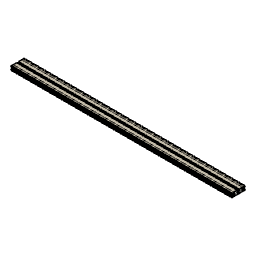
vector rail profile (Autodesk Fusion 360 design; units mm, degrees)
Autodesk Fusion 360 part; units mm, degrees
sketch "Sketch1" plane through (0, 0, 0) normal (1, 0, 0) x (0, 0, -1)
  line L0 (-12.7, -4.6736) -> (-12.7, -2.4765)
  line L1 (-12.7, -2.4765) -> (-10.8458, -2.4765)
  line L2 (-10.8458, -2.4765) -> (-10.8458, -3.556)
  line L3 (-10.8458, -3.556) -> (-8.2042, -3.556)
  line L4 (-8.2042, -3.556) -> (-8.2042, -2.4765)
  line L5 (-8.2042, -2.4765) -> (-6.9342, -2.4765)
  line L6 (-6.9342, -2.4765) -> (-6.9342, 0.5207)
  line L7 (-6.9342, 0.5207) -> (-8.2042, 0.5207)
  line L8 (-8.2042, 0.5207) -> (-8.2042, 1.6002)
  line L9 (-8.2042, 1.6002) -> (-10.8458, 1.6002)
  line L10 (-10.8458, 1.6002) -> (-10.8458, 0.5207)
  line L11 (-10.8458, 0.5207) -> (-12.7, 0.5207)
  line L12 (-12.7, 0.5207) -> (-12.7, 2.7178)
  line L13 (-12.7, 2.7178) -> (-1.4986, 2.7178)
  line L14 (-1.4986, 2.7178) -> (-1.4986, 1.3208)
  line L15 (-1.4986, 1.3208) -> (-2.5781, 1.3208)
  line L16 (-2.5781, 1.3208) -> (-2.5781, -1.3208)
  line L17 (-2.5781, -1.3208) -> (-1.4986, -1.3208)
  line L18 (-1.4986, -1.3208) -> (-1.4986, -2.5908)
  line L19 (-1.4986, -2.5908) -> (0, -2.5908)
  line L20 (0, -4.6736) -> (-12.7, -4.6736)
  line L21 (-9.525, -3.556) -> (-9.525, 1.6002) construction
  line L22 (0, -2.5908) -> (0, -4.6736)
  line L23 (-6.9342, -0.9779) -> (-13.037, -0.9779) construction
  line L24 (-2.5781, 0) -> (0, 0) construction
  dimension "d13" = 12.7
  dimension "d14" = 9.525
  dimension "d15" = 5.1562
  dimension "d16" = 7.3914
  dimension "d17" = 1.27
  dimension "d18" = 2.6416
  dimension "d19" = 1.8542
  dimension "d20" = 2.9972
  dimension "d21" = 1.1176
  dimension "d22" = 1.397
  dimension "d23" = 2.5781
  dimension "d24" = 2.6416
  dimension "d25" = 1.27
  dimension "d26" = 1.4986
  constraint vertical L0
  constraint perpendicular L0 L1
  constraint perpendicular L1 L2
  constraint perpendicular L2 L3
  constraint perpendicular L3 L4
  constraint perpendicular L4 L5
  constraint perpendicular L5 L6
  constraint perpendicular L6 L7
  constraint perpendicular L7 L8
  constraint perpendicular L2 L9
  constraint perpendicular L9 L10
  constraint perpendicular L0 L11
  constraint perpendicular L1 L12
  constraint perpendicular L0 L13
  constraint perpendicular L1 L14
  constraint perpendicular L0 L15
  constraint perpendicular L15 L16
  constraint perpendicular L14 L17
  constraint perpendicular L17 L18
  constraint perpendicular L14 L19
  constraint horizontal L20
  constraint collinear L14 L18
  constraint collinear L4 L8
  constraint collinear L2 L10
  constraint collinear L7 L11
  constraint collinear L1 L5
  constraint midpoint L3 L21.start
  constraint midpoint L9 L21.end
  constraint perpendicular L20 L22
  constraint midpoint L6 L23.start
  constraint perpendicular L21 L23
  constraint symmetric L3 L9 L23
  constraint midpoint L16 L24.start
  constraint perpendicular L22 L24
  constraint coincident L20.start L22.end
  constraint coincident L24.end origin
  constraint vertical L24.end L19.end
  measures "d13" distance of L0 L22
  measures "d14" distance of L21 L22
  measures "d15" distance of L3 L9
  measures "d16" distance of L13 L20
  measures "d17" distance of L6 L8
  measures "d18" distance of L8 L10
  measures "d19" distance of L10 L12
  measures "d20" distance of L1 L11
  measures "d21" distance of L3 L20
  measures "d22" distance of L13 L15
  measures "d23" distance of L16 L22
  measures "d24" distance of L15.end L16.end
  measures "d25" distance of L17 L19
  measures "d26" distance of L18 L22
extrude "Extrude1" add sketch "Sketch1" along normal blind 426.72 makes body 1
mirror "Mirror1" about plane through (0, 0, 0) normal (0, 0, 1) of bodies 1 makes body 2
combine "Combine1" operation add target body 1 tool bodies 2
equation "d13 = ( 1 / 2 ) * 1 in"
equation "d14 = ( 0.75 / 2 ) * 1 in"
equation "d23 = ( 0.203 / 2 ) * 1 in"
equation "d26 = ( 0.118 / 2 ) * 1 in"
equation "hp_length = 84"
equation "hp_constant = 5.08 mm"
equation "d29 = hp_constant * hp_length"
